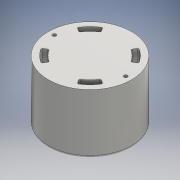
# Autodesk Inventor part: middle orbit
Saved by Autodesk Inventor 2016 (Build 200138000, 138)
## iProperties
Created: 2016-04-26
Part Number: middle orbit
Material: ABS Plastic
Document SubType Name: Modeling
Designer: Hamid Osooli
Density: 1.06 g/cm^3
Appearance: Smooth - White
Mass: 173.221 g
Surface Area: 257.563 cm^2
Volume: 163.416 cm^3
Author: Hamid Osooli
Autodesk Inventor part; units mm, degrees
ref_plane "YZ Plane" through (0, 0, 0) normal (1, 0, 0) x (0, 1, 0)
ref_plane "XZ Plane" through (0, 0, 0) normal (0, 1, 0) x (-1, 0, 0)
ref_plane "XY Plane" through (0, 0, 0) normal (0, 0, 1) x (1, 0, 0)
sketch "Sketch1" plane through (0, 0, 0) normal (0, 0, 1) x (1, 0, 0)
  circle A0 centre (0, 0) radius 35
  dimension "d0" = 70
  constraints: 1 centre point, 1 coincident
  measures "d0" diameter of A0
extrude "Extrusion1" add sketch "Sketch1" along normal blind 50
sketch "Sketch4" plane through (0, 0, 50) normal (0, 0, 1) x (1, 0, 0)
  circle A0 centre (30, 0) radius 1.5
  dimension "d104" = 3
  constraints: 1 centre point
  measures "d104" diameter of A0
sketch "Sketch6" plane through (0, 0, 50) normal (0, 0, 1) x (1, 0, 0)
  circle A0 centre (-30, 0) radius 1.5
  point P0 (0, 0)
  dimension "d105" = 3
  constraints: 1 centre point
  measures "d105" diameter of A0
sketch "Sketch11" plane through (0, 0, 0) normal (0, 0, -1) x (-1, 0, 0)
  line L0 (13.8079, 12.25) -> (-13.8079, 12.25)
  line L1 (-18.25, 8.6641) -> (-18.25, -8.6641)
  line L2 (-13.8079, -12.25) -> (13.8079, -12.25)
  line L3 (18.25, -8.6641) -> (18.25, 8.6641)
  line L4 (17.3393, 10.3414) -> (14.8972, 11.9273)
  line L5 (17.3393, -10.3414) -> (14.8972, -11.9273)
  line L6 (-17.3393, 10.3414) -> (-14.8972, 11.9273)
  line L7 (-17.3393, -10.3414) -> (-14.8972, -11.9273)
  arc A0 (18.25, 8.6641) -> (17.3393, 10.3414) centre (16.25, 8.6641) ccw
  arc A1 (14.8972, 11.9273) -> (13.8079, 12.25) centre (13.8079, 10.25) ccw
  arc A2 (17.3393, -10.3414) -> (18.25, -8.6641) centre (16.25, -8.6641) ccw
  arc A3 (13.8079, -12.25) -> (14.8972, -11.9273) centre (13.8079, -10.25) ccw
  arc A4 (-14.8972, -11.9273) -> (-13.8079, -12.25) centre (-13.8079, -10.25) ccw
  arc A5 (-18.25, -8.6641) -> (-17.3393, -10.3414) centre (-16.25, -8.6641) ccw
  arc A6 (-17.3393, 10.3414) -> (-18.25, 8.6641) centre (-16.25, 8.6641) ccw
  arc A7 (-13.8079, 12.25) -> (-14.8972, 11.9273) centre (-13.8079, 10.25) ccw
  point P0 (18.25, 12.25)
  point P1 (-18.25, -12.25)
  point P2 (-18.25, 12.25)
  point P3 (18.25, -12.25)
  point P4 (18.25, 9.75)
  point P5 (18.25, -9.75)
  point P6 (-18.25, 9.75)
  point P7 (-18.25, -9.75)
  dimension "d73" = 36.5
  dimension "d74" = 24.5
  dimension "d75" = 2.5
  dimension "d76" = 57
  dimension "d77" = 2.5
  dimension "d78" = 57
  dimension "d79" = 2.5
  dimension "d80" = 57
  dimension "d81" = 2.5
  dimension "d82" = 57
  dimension "d83" = 2
  constraints: 16 end point, 16 point on circle, 16 point on line, 16 tangent, 8 centre point, 7 equal radius, 2 parallel, 1 horizontal, 1 perpendicular
  measures "d73" distance of point (18.25, -12.25) point (-18.25, -12.25)
  measures "d74" distance of point (-18.25, -12.25) point (-18.25, 12.25)
  measures "d75" distance of point (18.25, 9.75) point (18.25, 12.25)
  measures "d76" angle of L3 L4
  measures "d77" distance of point (18.25, -9.75) point (18.25, -12.25)
  measures "d78" angle of L3 L5
  measures "d79" distance of point (-18.25, 9.75) point (-18.25, 12.25)
  measures "d80" angle of L1 L6
  measures "d81" distance of point (-18.25, -9.75) point (-18.25, -12.25)
  measures "d82" angle of L1 L7
  measures "d83" radius of A0
extrude "Extrusion2" cut sketch "Sketch11" against normal blind 27.5
sketch "Sketch12" plane through (0, 0, 50) normal (0, 0, 1) x (1, 0, 0)
  line L0 (0, 0) -> (30, 0) construction
  line L1 (0, 0) -> (30, 0) construction
  arc A0 (-12.5, 21.6506) -> (-21.6506, 12.5) centre (0, 0) ccw
  arc A1 (-15, 25.9808) -> (-25.9808, 15) centre (0, 0) ccw
  arc A2 (25.9808, 15) -> (15, 25.9808) centre (0, 0) ccw
  arc A3 (21.6506, 12.5) -> (12.5, 21.6506) centre (0, 0) ccw
  arc A4 (15, -25.9808) -> (25.9808, -15) centre (0, 0) ccw
  arc A5 (12.5, -21.6506) -> (21.6506, -12.5) centre (0, 0) ccw
  arc A6 (-21.6506, -12.5) -> (-12.5, -21.6506) centre (0, 0) ccw
  arc A7 (-25.9808, -15) -> (-15, -25.9808) centre (0, 0) ccw
  line L2 (-21.6506, 12.5) -> (-25.9808, 15)
  line L3 (-12.5, 21.6506) -> (-15, 25.9808)
  line L4 (12.5, 21.6506) -> (15, 25.9808)
  line L5 (21.6506, 12.5) -> (25.9808, 15)
  line L6 (25.9808, -15) -> (21.6506, -12.5)
  line L7 (15, -25.9808) -> (12.5, -21.6506)
  line L8 (-12.5, -21.6506) -> (-15, -25.9808)
  line L9 (-21.6506, -12.5) -> (-25.9808, -15)
  constraints: 20 end point, 17 point on circle, 8 centre point, 6 perpendicular, 2 horizontal
extrude "Extrusion3" cut sketch "Sketch12" against normal blind 10
fillet "Fillet3" radius 2 1 edges at (-35, 0, 0)
fillet "Fillet6" radius 1 16 edges at (12.5, 21.6506, 45) (21.6506, 12.5, 45) (25.9808, 15, 45) (15, 25.9808, 45) (-15, 25.9808, 45) (-12.5, 21.6506, 45) (-21.6506, 12.5, 45) (-25.9808, 15, 45) (-21.6506, -12.5, 45) (-25.9808, -15, 45) (-15, -25.9808, 45) (-12.5, -21.6506, 45) (12.5, -21.6506, 45) (15, -25.9808, 45) (25.9808, -15, 45) (21.6506, -12.5, 45)
sketch "Sketch15" plane through (0, 0, 27.5) normal (0, 0, -1) x (-1, 0, 0)
  circle A0 centre (-15.25, 0) radius 1.75
  circle A1 centre (-15.25, -6.5) radius 1.75
  circle A2 centre (-15.25, 6.5) radius 1.75
  point P0 (0, 0)
  dimension "d85" = 3.5
  constraints: 3 centre point
  measures "d85" diameter of A0
extrude "Extrusion6" add sketch "Sketch15" along normal blind 24
sketch "Sketch16" plane through (0, 0, 0) normal (0, 0, -1) x (-1, 0, 0)
  line L0 (-8, 23) -> (8, 23)
  line L1 (10, 21) -> (10, 20)
  line L2 (8, 18) -> (-8, 18)
  line L3 (-10, 20) -> (-10, 21)
  arc A0 (21.1538, 13.3235) -> (13.3235, 21.1538) centre (0, 0) ccw projected
  line L4 (8, -18) -> (-7.798, -18)
  line L5 (-9.798, -20) -> (-9.798, -21)
  line L6 (-7.798, -23) -> (8, -23)
  line L7 (10, -21) -> (10, -20)
  arc A1 (10, 21) -> (8, 23) centre (8, 21) ccw
  arc A2 (8, 18) -> (10, 20) centre (8, 20) ccw
  arc A3 (-10, 20) -> (-8, 18) centre (-8, 20) ccw
  arc A4 (-8, 23) -> (-10, 21) centre (-8, 21) ccw
  arc A5 (-7.798, -18) -> (-9.798, -20) centre (-7.798, -20) ccw
  arc A6 (10, -20) -> (8, -18) centre (8, -20) ccw
  arc A7 (8, -23) -> (10, -21) centre (8, -21) ccw
  arc A8 (-9.798, -21) -> (-7.798, -23) centre (-7.798, -21) ccw
  point P0 (0, 0)
  point P1 (10, 18)
  point P2 (10, 23)
  point P3 (-10, 18)
  point P4 (10, -18)
  point P5 (-9.798, -23)
  point P6 (-9.798, -18)
  dimension "d90" = 20
  dimension "d91" = 5
  dimension "d92" = 5
  dimension "d93" = 2
  constraints: 17 point on circle, 16 end point, 16 tangent, 13 point on line, 8 centre point, 7 equal radius, 4 parallel, 2 horizontal, 2 perpendicular
  measures "d90" distance of point (10, 18) point (-10, 18)
  measures "d91" distance of point (10, 23) point (10, 18)
  measures "d92" distance of point (-9.798, -23) point (-9.798, -18)
  measures "d93" radius of A1
extrude "Extrusion7" cut sketch "Sketch16" against normal blind 10
extrude "Extrusion10" cut sketch "Sketch6" against normal through all
extrude "Extrusion11" cut sketch "Sketch4" against normal through all
equation "\"d77\" = d75"
equation "\"d78\" = d76"
body "Solid1"
